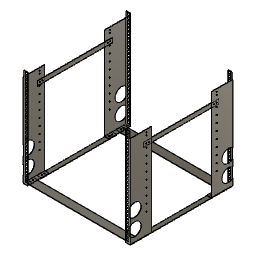
TV Cabinet Rack Posts (Autodesk Fusion 360 design; units mm, degrees)
Autodesk Fusion 360 part; units mm, degrees
sketch "Sketch1" plane through (0, 0, 0) normal (1, 0, 0) x (0, 1, 0) in component "Rack Postst"
  line L0 (-75, 0) -> (24, 0)
  line L1 (24, 0) -> (24, 425)
  line L2 (24, 425) -> (-75, 425)
  line L3 (-75, 425) -> (-75, 0)
  line L4 (0, 1.75) -> (0, 22.5)
  circle A0 centre (-54, 53) radius 30
  circle A1 centre (-54, 130) radius 30
  circle A2 centre (0, 96) radius 2.5
  circle A3 centre (0, 128) radius 2.5
  circle A4 centre (0, 160) radius 2.5
  circle A5 centre (0, 192) radius 2.5
  circle A6 centre (0, 224) radius 2.5
  circle A7 centre (0, 256) radius 2.5
  circle A8 centre (0, 288) radius 2.5
  circle A9 centre (0, 320) radius 2.5
  circle A10 centre (0, 352) radius 2.5
  circle A11 centre (0, 413) radius 2.5
  circle A12 centre (0, 401) radius 2.5
  circle A13 centre (0, 369) radius 2.5
  circle A14 centre (12, 369) radius 2.5
  dimension "d1017" = 75
  dimension "d1018" = 24
  dimension "d1019" = 425
  dimension "d1020" = 60
  dimension "d1021" = 53
  dimension "d1022" = 54
  dimension "d1025" = 0
  dimension "d1026" = 77
  dimension "d1033" = 5
  dimension "d1034" = 96
  dimension "d1037" = 0
  dimension "d1038" = 32
  dimension "d1152" = 5
  dimension "d1153" = 12
  dimension "d1156" = 0
  dimension "d1157" = -12
  dimension "d1158" = 5
  dimension "d1159" = 32
  dimension "d1162" = 12
  dimension "d1163" = 0
  constraint horizontal L0
  constraint vertical L1
  constraint horizontal L2
  constraint vertical L3
  constraint coincident origin L0
  measures "d1017" distance of L3 L4
  measures "d1018" distance of L1 L4
  measures "d1019" distance of origin L2
  measures "d1020" diameter of A0
  measures "d1021" distance of L0 A0.centre
  measures "d1022" distance of L4 A0.centre
  measures "d1033" diameter of A2
  measures "d1034" distance of origin A2.centre
  measures "d1152" diameter of A11
  measures "d1153" distance of L2 A11.centre
  measures "d1158" diameter of A13
  measures "d1159" distance of A12.centre A13.centre
extrude "Extrude1" add sketch "Sketch1" along normal blind 1.98 contours L0 L1 L2 L3 A0 A1 makes body 1 in component "Rack Postst"
sketch "Sketch2" plane through (0, -75, 0) normal (0, -1, 0) x (1, 0, 0) in component "Rack Postst"
  line L0 (0, 425) -> (0, 151.4243)
  line L1 (0, 151.4243) -> (1.98, 151.4243)
  line L2 (1.98, 151.4243) -> (1.98, 425)
  line L3 (1.98, 425) -> (0, 425)
  line L4 (1.98, 454) -> (22, 454)
  line L5 (22, 454) -> (22, 0)
  line L6 (22, 0) -> (1.98, 0)
  line L7 (1.98, 0) -> (1.98, 454)
  line L8 (1.98, 454) -> (3, 454)
  line L9 (3, 454) -> (3, 425)
  line L10 (3, 425) -> (1.98, 425)
  line L11 (1.98, 425) -> (1.98, 454)
  line L12 (19.75, 450.8) -> (10.25, 450.8)
  line L13 (10.25, 450.8) -> (10.25, 441.3)
  line L14 (10.25, 441.3) -> (19.75, 441.3)
  line L15 (19.75, 441.3) -> (19.75, 450.8)
  line L16 (19.75, 434.925) -> (10.25, 434.925)
  line L17 (10.25, 434.925) -> (10.25, 425.425)
  line L18 (10.25, 425.425) -> (19.75, 425.425)
  line L19 (19.75, 425.425) -> (19.75, 434.925)
  line L20 (19.75, 419.05) -> (10.25, 419.05)
  line L21 (10.25, 419.05) -> (10.25, 409.55)
  line L22 (10.25, 409.55) -> (19.75, 409.55)
  line L23 (19.75, 409.55) -> (19.75, 419.05)
  line L24 (19.75, 396.85) -> (19.75, 406.35)
  line L25 (10.25, 396.85) -> (19.75, 396.85)
  line L26 (10.25, 406.35) -> (10.25, 396.85)
  line L27 (19.75, 406.35) -> (10.25, 406.35)
  line L28 (19.75, 390.475) -> (10.25, 390.475)
  line L29 (19.75, 380.975) -> (19.75, 390.475)
  line L30 (10.25, 380.975) -> (19.75, 380.975)
  line L31 (10.25, 390.475) -> (10.25, 380.975)
  line L32 (19.75, 374.6) -> (10.25, 374.6)
  line L33 (19.75, 365.1) -> (19.75, 374.6)
  line L34 (10.25, 365.1) -> (19.75, 365.1)
  line L35 (10.25, 374.6) -> (10.25, 365.1)
  line L36 (19.75, 352.4) -> (19.75, 361.9)
  line L37 (10.25, 352.4) -> (19.75, 352.4)
  line L38 (10.25, 361.9) -> (10.25, 352.4)
  line L39 (19.75, 361.9) -> (10.25, 361.9)
  line L40 (19.75, 346.025) -> (10.25, 346.025)
  line L41 (19.75, 336.525) -> (19.75, 346.025)
  line L42 (10.25, 336.525) -> (19.75, 336.525)
  line L43 (10.25, 346.025) -> (10.25, 336.525)
  line L44 (19.75, 330.15) -> (10.25, 330.15)
  line L45 (19.75, 320.65) -> (19.75, 330.15)
  line L46 (10.25, 320.65) -> (19.75, 320.65)
  line L47 (10.25, 330.15) -> (10.25, 320.65)
  line L48 (19.75, 307.95) -> (19.75, 317.45)
  line L49 (10.25, 307.95) -> (19.75, 307.95)
  line L50 (10.25, 317.45) -> (10.25, 307.95)
  line L51 (19.75, 317.45) -> (10.25, 317.45)
  line L52 (19.75, 301.575) -> (10.25, 301.575)
  line L53 (19.75, 292.075) -> (19.75, 301.575)
  line L54 (10.25, 292.075) -> (19.75, 292.075)
  line L55 (10.25, 301.575) -> (10.25, 292.075)
  line L56 (19.75, 285.7) -> (10.25, 285.7)
  line L57 (19.75, 276.2) -> (19.75, 285.7)
  line L58 (10.25, 276.2) -> (19.75, 276.2)
  line L59 (10.25, 285.7) -> (10.25, 276.2)
  line L60 (19.75, 263.5) -> (19.75, 273)
  line L61 (10.25, 263.5) -> (19.75, 263.5)
  line L62 (10.25, 273) -> (10.25, 263.5)
  line L63 (19.75, 273) -> (10.25, 273)
  line L64 (19.75, 257.125) -> (10.25, 257.125)
  line L65 (19.75, 247.625) -> (19.75, 257.125)
  line L66 (10.25, 247.625) -> (19.75, 247.625)
  line L67 (10.25, 257.125) -> (10.25, 247.625)
  line L68 (19.75, 241.25) -> (10.25, 241.25)
  line L69 (19.75, 231.75) -> (19.75, 241.25)
  line L70 (10.25, 231.75) -> (19.75, 231.75)
  line L71 (10.25, 241.25) -> (10.25, 231.75)
  line L72 (19.75, 219.05) -> (19.75, 228.55)
  line L73 (10.25, 219.05) -> (19.75, 219.05)
  line L74 (10.25, 228.55) -> (10.25, 219.05)
  line L75 (19.75, 228.55) -> (10.25, 228.55)
  line L76 (19.75, 212.675) -> (10.25, 212.675)
  line L77 (19.75, 203.175) -> (19.75, 212.675)
  line L78 (10.25, 203.175) -> (19.75, 203.175)
  line L79 (10.25, 212.675) -> (10.25, 203.175)
  line L80 (19.75, 196.8) -> (10.25, 196.8)
  line L81 (19.75, 187.3) -> (19.75, 196.8)
  line L82 (10.25, 187.3) -> (19.75, 187.3)
  line L83 (10.25, 196.8) -> (10.25, 187.3)
  line L84 (19.75, 174.6) -> (19.75, 184.1)
  line L85 (10.25, 174.6) -> (19.75, 174.6)
  line L86 (10.25, 184.1) -> (10.25, 174.6)
  line L87 (19.75, 184.1) -> (10.25, 184.1)
  line L88 (19.75, 168.225) -> (10.25, 168.225)
  line L89 (19.75, 158.725) -> (19.75, 168.225)
  line L90 (10.25, 158.725) -> (19.75, 158.725)
  line L91 (10.25, 168.225) -> (10.25, 158.725)
  line L92 (19.75, 152.35) -> (10.25, 152.35)
  line L93 (19.75, 142.85) -> (19.75, 152.35)
  line L94 (10.25, 142.85) -> (19.75, 142.85)
  line L95 (10.25, 152.35) -> (10.25, 142.85)
  line L96 (19.75, 130.15) -> (19.75, 139.65)
  line L97 (10.25, 130.15) -> (19.75, 130.15)
  line L98 (10.25, 139.65) -> (10.25, 130.15)
  line L99 (19.75, 139.65) -> (10.25, 139.65)
  line L100 (19.75, 123.775) -> (10.25, 123.775)
  line L101 (19.75, 114.275) -> (19.75, 123.775)
  line L102 (10.25, 114.275) -> (19.75, 114.275)
  line L103 (10.25, 123.775) -> (10.25, 114.275)
  line L104 (19.75, 107.9) -> (10.25, 107.9)
  line L105 (19.75, 98.4) -> (19.75, 107.9)
  line L106 (10.25, 98.4) -> (19.75, 98.4)
  line L107 (10.25, 107.9) -> (10.25, 98.4)
  line L108 (19.75, 85.7) -> (19.75, 95.2)
  line L109 (10.25, 85.7) -> (19.75, 85.7)
  line L110 (10.25, 95.2) -> (10.25, 85.7)
  line L111 (19.75, 95.2) -> (10.25, 95.2)
  line L112 (19.75, 79.325) -> (10.25, 79.325)
  line L113 (19.75, 69.825) -> (19.75, 79.325)
  line L114 (10.25, 69.825) -> (19.75, 69.825)
  line L115 (10.25, 79.325) -> (10.25, 69.825)
  line L116 (19.75, 63.45) -> (10.25, 63.45)
  line L117 (19.75, 53.95) -> (19.75, 63.45)
  line L118 (10.25, 53.95) -> (19.75, 53.95)
  line L119 (10.25, 63.45) -> (10.25, 53.95)
  line L120 (19.75, 41.25) -> (19.75, 50.75)
  line L121 (10.25, 41.25) -> (19.75, 41.25)
  line L122 (10.25, 50.75) -> (10.25, 41.25)
  line L123 (19.75, 50.75) -> (10.25, 50.75)
  line L124 (19.75, 34.875) -> (10.25, 34.875)
  line L125 (19.75, 25.375) -> (19.75, 34.875)
  line L126 (10.25, 25.375) -> (19.75, 25.375)
  line L127 (10.25, 34.875) -> (10.25, 25.375)
  line L128 (19.75, 19) -> (10.25, 19)
  line L129 (19.75, 9.5) -> (19.75, 19)
  line L130 (10.25, 9.5) -> (19.75, 9.5)
  line L131 (10.25, 19) -> (10.25, 9.5)
  point P0 (1.98, 0)
  dimension "d1041" = 22
  dimension "d1042" = 454
  dimension "d1043" = 3
  dimension "d1044" = 425
  dimension "d1045" = 9.5
  dimension "d1046" = 9.5
  dimension "d1047" = 2.25
  dimension "d1048" = 3.2
  dimension "d1051" = 0
  dimension "d1052" = -15.875
  dimension "d1055" = 0
  dimension "d1056" = -44.45
  constraint horizontal L4
  constraint vertical L5
  constraint horizontal L6
  constraint vertical L7
  constraint coincident L2 L4.start
  constraint coincident L6 P0
  constraint horizontal L8
  constraint vertical L9
  constraint horizontal L10
  constraint vertical L11
  constraint horizontal L12
  constraint vertical L13
  constraint horizontal L14
  constraint vertical L15
  measures "d1041" distance of L0 L5
  measures "d1042" distance of L4 L6
  measures "d1043" distance of L0 L9
  measures "d1044" distance of P0 L10
  measures "d1045" distance of L12.start L12.end
  measures "d1046" distance of L12.start L14.end
  measures "d1047" distance of L5 L15
  measures "d1048" distance of L4 L12
extrude "Extrude2" add sketch "Sketch2" against normal blind 1.98 contours L2 L4 L5 L6 L7 L9 L10 bodies 1 in component "Rack Postst"
sketch "Sketch3" plane through (0, 0, 0) normal (0, 0, -1) x (1, 0, 0) in component "Rack Postst"
  line L0 (0, 75) -> (0, -24)
  line L1 (0, -24) -> (1.98, -24)
  line L2 (1.98, -24) -> (1.98, 73.02)
  line L3 (1.98, 73.02) -> (22, 73.02)
  line L4 (22, 73.02) -> (22, 75)
  line L5 (22, 75) -> (0, 75)
  line L6 (1.98, -24) -> (22, -24)
  line L7 (22, -24) -> (22, 65)
  line L8 (22, 65) -> (1.98, 65)
  line L9 (1.98, 65) -> (1.98, -24)
  circle A0 centre (12, 53) radius 2.5
  circle A1 centre (12, -12) radius 2.5
  circle A2 centre (12, 41) radius 2.5
  circle A3 centre (12, 0) radius 2.5
  dimension "d1059" = 65
  dimension "d1060" = 5
  dimension "d1061" = 12
  dimension "d1062" = 5
  dimension "d1063" = 12
  dimension "d1064" = 10
  dimension "d1065" = 10
  dimension "d1068" = 0
  dimension "d1069" = -12
  dimension "d1072" = 0
  dimension "d1073" = 12
  constraint horizontal L6
  constraint vertical L7
  constraint horizontal L8
  constraint vertical L9
  constraint coincident L1.end L2.start
  constraint coincident L3.end L7
  measures "d1059" distance of origin L8
  measures "d1060" diameter of A0
  measures "d1061" distance of L8 A0.centre
  measures "d1062" diameter of A1
  measures "d1063" distance of L6 A1.centre
  measures "d1064" distance of L7 A0.centre
  measures "d1065" distance of L7 A1.centre
extrude "Extrude3" add sketch "Sketch3" against normal blind 1.98 contours L2 L6 L7 L8 L9 bodies 1 in component "Rack Postst"
ref_plane "WorkPlane1" through (247.5, 0, 0) normal (1, 0, 0) x (0, 1, 0) in component "Rack Postst"
mirror "Mirror4" about plane through (247.5, 0, 0) normal (1, 0, 0) of bodies 1 makes body 2 in component "Rack Postst"
ref_plane "WorkPlane2" through (0, 162, 0) normal (0, 1, 0) x (0, 0, 1) in component "Rack Postst"
mirror "Mirror5" about plane through (0, 162, 0) normal (0, 1, 0) of bodies 2 1 makes body 3 at (0, 373.7148, 289.0876) makes body 4 at (495, 373.7148, 289.0876) in component "Rack Postst"
sketch "Sketch1 (2)" plane through (0, 0, 0) normal (0, 0, 1) x (1, 0, 0) in component "Bracing"
  line L0 (493, -65.5) -> (2, -65.5)
  line L1 (2, -65.5) -> (2, -28.5)
  line L2 (2, -28.5) -> (493, -28.5)
  line L3 (493, -28.5) -> (493, -65.5)
  line L4 (495, -75) -> (495, 24)
  circle A0 centre (483, -53) radius 2.5
  circle A1 centre (483, -41) radius 2.5
  line L5 (0, -75) -> (0, 24)
  circle A2 centre (483, -53) radius 2.5
  circle A3 centre (483, -41) radius 2.5
  circle A4 centre (12, -53) radius 2.5
  circle A5 centre (12, -41) radius 2.5
  point P0 (12, -53)
  point P1 (12, -41)
  dimension "d1170" = 2
  dimension "d1171" = 12.5
  dimension "d1172" = 12.5
  dimension "d1173" = 2
  dimension "d1174" = 5
  dimension "d1175" = 5
  dimension "d1176" = 5
  dimension "d1177" = 5
  constraint horizontal L0
  constraint vertical L1
  constraint horizontal L2
  constraint vertical L3
  constraint concentric A0 A2
  constraint concentric A1 A3
  constraint coincident P0 A4.centre
  constraint coincident P1 A5.centre
  measures "d1170" distance of L3 L4
  measures "d1171" distance of L0 A0.centre
  measures "d1172" distance of L2 A1.centre
  measures "d1173" distance of L1 L5
  measures "d1174" diameter of A2
  measures "d1175" diameter of A3
  measures "d1176" diameter of A4
  measures "d1177" diameter of A5
extrude "Extrude1'" add sketch "Sketch1 (2)" against normal blind 1.98 separate body makes body 5 in component "Bracing"
mirror "Mirror1" about plane through (0, 162, 0) normal (0, 1, 0) of bodies 5 makes body 6 in component "Bracing"
sketch "Sketch2 (2)" plane through (0, 0, 0) normal (0, 0, 1) x (1, 0, 0) in component "Bracing"
  line L0 (493, -12) -> (473, -12)
  line L1 (473, -12) -> (473, 336)
  line L2 (473, 336) -> (493, 336)
  line L3 (493, 336) -> (493, -12)
  circle A0 centre (483, 0) radius 2.5
  circle A1 centre (483, 324) radius 2.5
  circle A2 centre (483, 0) radius 2.5
  circle A3 centre (483, 324) radius 2.5
  circle A4 centre (483, 312) radius 2.5
  circle A5 centre (483, 12) radius 2.5
  dimension "d1181" = 10
  dimension "d1182" = 10
  dimension "d1183" = 12
  dimension "d1184" = 12
  dimension "d1185" = 5
  dimension "d1186" = 5
  dimension "d1187" = 5
  dimension "d1188" = 12
  dimension "d1189" = 5
  dimension "d1190" = 12
  constraint horizontal L0
  constraint vertical L1
  constraint horizontal L2
  constraint vertical L3
  constraint concentric A0 A2
  constraint concentric A1 A3
  measures "d1181" distance of L1 A0.centre
  measures "d1182" distance of L3 A0.centre
  measures "d1183" distance of L0 A0.centre
  measures "d1184" distance of L2 A1.centre
  measures "d1185" diameter of A2
  measures "d1186" diameter of A3
  measures "d1187" diameter of A4
  measures "d1188" distance of A1.centre A4.centre
  measures "d1189" diameter of A5
  measures "d1190" distance of A0.centre A5.centre
extrude "Extrude2'" add sketch "Sketch2 (2)" against normal blind 1.98 separate body makes body 7 in component "Bracing"
mirror "Mirror2" about plane through (247.5, 0, 0) normal (1, 0, 0) of bodies 7 makes body 8 in component "Bracing"
copy_body "CopyPasteBodies1" bodies 8 makes body 9 in component "Bracing"
move_body "Move1" bodies 9 to x (0, 0, -1) y (0, 1, 0) z (1, 0, 0) at (12.2483, 0, 12.2483) in component "Bracing"
move_body "Align1" bodies 9 to x (1, 0, 0) y (0, 1, 0) z (0, 0, 1) at (-8.2883, 0, 368.7517) in component "Bracing"
mirror "Mirror3" about plane through (247.5, 0, 0) normal (1, 0, 0) of bodies 9 makes body 10 in component "Bracing"
component "Rack Postst" placed x (1, 0, 0) y (0, 1, 0) z (0, 0, 1) at (0, 0, 0)
component "Bracing" placed x (1, 0, 0) y (0, 1, 0) z (0, 0, 1) at (0, 0, 0)
named bodies: "FL Post", "FR Post", "BL Post", "BR Post", "LR Front", "LR Rear", "FB Right", "FB Left", "FB Left Top", "FB Right Top"
